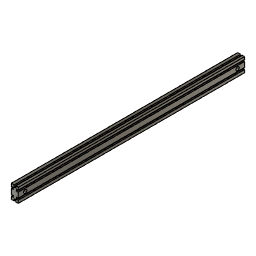
clearbot v9 (Autodesk Fusion 360 archive; units mm, degrees)
design "40X80X1300_AlBar"
Autodesk Fusion 360 part; units mm, degrees
sketch "Sketch1" plane through (0, 0, 0) normal (0, 1, 0) x (1, 0, 0)
  line L0 (20, -40) -> (-20, 40) construction
  line L1 (-20, -40) -> (20, 40) construction
  line L2 (5, 29) -> (-5, 29)
  line L3 (-5, 29) -> (-5, 39)
  line L4 (5, 39) -> (5, 29)
  line L5 (5, 29) -> (-5, 39) construction
  line L6 (-5, 29) -> (5, 39) construction
  line L7 (-4, 39) -> (-4, 40)
  line L8 (4, 39) -> (4, 40)
  line L9 (-19, 25) -> (-9, 25)
  line L10 (-9, 25) -> (-9, 15)
  line L11 (-9, 15) -> (-19, 15)
  line L12 (19, 25) -> (9, 25)
  line L13 (9, 25) -> (9, 15)
  line L14 (9, 15) -> (19, 15)
  line L15 (-20, 16) -> (-19, 16)
  line L16 (-19, 24) -> (-20, 24)
  line L17 (19, 16) -> (20, 16)
  line L18 (20, 24) -> (19, 24)
  line L19 (-20, 24) -> (-20, 40)
  line L20 (-19, 15) -> (-19, 16)
  line L21 (-19, 24) -> (-19, 25)
  line L22 (19, 15) -> (19, 16)
  line L23 (19, 24) -> (19, 25)
  line L24 (-20, 40) -> (-4, 40)
  line L25 (4, 40) -> (20, 40)
  line L26 (-5, 39) -> (-4, 39)
  line L27 (4, 39) -> (5, 39)
  line L28 (20, 40) -> (20, 24)
  line L29 (1.75, 0) -> (22.5, 0)
  line L30 (-19, -24) -> (-20, -24)
  line L31 (-19, -24) -> (-19, -25)
  line L32 (-19, -25) -> (-9, -25)
  line L33 (-20, -16) -> (-19, -16)
  line L34 (-19, -15) -> (-19, -16)
  line L35 (-9, -15) -> (-19, -15)
  line L36 (-9, -25) -> (-9, -15)
  line L37 (-4, -39) -> (-4, -40)
  line L38 (-5, -39) -> (-4, -39)
  line L39 (-5, -29) -> (-5, -39)
  line L40 (5, -29) -> (-5, -29)
  line L41 (5, -39) -> (5, -29)
  line L42 (4, -39) -> (5, -39)
  line L43 (4, -39) -> (4, -40)
  line L44 (20, -24) -> (19, -24)
  line L45 (19, -24) -> (19, -25)
  line L46 (19, -25) -> (9, -25)
  line L47 (9, -25) -> (9, -15)
  line L48 (9, -15) -> (19, -15)
  line L49 (19, -15) -> (19, -16)
  line L50 (19, -16) -> (20, -16)
  line L51 (-20, -40) -> (-20, -24)
  line L52 (-20, -16) -> (-20, 16)
  line L53 (20, 16) -> (20, -16)
  line L54 (20, -24) -> (20, -40)
  line L55 (20, -40) -> (4, -40)
  line L56 (-4, -40) -> (-20, -40)
  point P0 (0, 34)
  dimension "d20" = 40
  dimension "d21" = 80
  dimension "d22" = 10
  dimension "d23" = 10
  dimension "d24" = 20
  dimension "d25" = 16
  dimension "d26" = 16
  dimension "d27" = 1
  dimension "d28" = 15
  dimension "d29" = 15
  dimension "d30" = 10
  dimension "d31" = 10
  dimension "d32" = 10
  dimension "d33" = 10
  dimension "d34" = 16
  dimension "d35" = 8
  dimension "d36" = 1
  dimension "d37" = 16
  dimension "d38" = 8
  dimension "d39" = 1
  constraint horizontal L55
  constraint perpendicular L51 L55
  constraint parallel L24 L55
  constraint parallel L28 L51
  constraint coincident L0 origin
  constraint coincident L1 origin
  constraint horizontal L2
  constraint perpendicular L2 L3
  constraint parallel L2 L26
  constraint parallel L3 L4
  constraint coincident L5 P0
  constraint coincident L6 P0
  constraint perpendicular L7 L24
  constraint coincident L8.start L26
  constraint coincident L8.end L24
  constraint perpendicular L8 L24
  constraint horizontal L9
  constraint vertical L10
  constraint horizontal L11
  constraint vertical L20
  constraint horizontal L12
  constraint vertical L13
  constraint horizontal L14
  constraint vertical L22
  constraint perpendicular L15 L20
  constraint coincident L16.start L20
  constraint coincident L16.end L51
  constraint perpendicular L16 L51
  constraint coincident L17.end L28
  constraint perpendicular L17 L28
  constraint coincident L18.end L22
  constraint perpendicular L18 L22
  constraint collinear L19 L51
  constraint collinear L20 L21
  constraint collinear L22 L23
  constraint collinear L24 L25
  constraint collinear L26 L27
  constraint collinear L28 L53
  constraint symmetric L2.start L29 L40.start
  constraint symmetric L2.end L29 L39.start
  constraint symmetric L3.end L29 L38.start
  constraint symmetric L4.start L29 L41.start
  constraint symmetric L7.start L29 L37.start
  constraint symmetric L7.end L29 L37.end
  constraint symmetric L8.start L29 L42.start
  constraint symmetric L8.end L29 L43.end
  constraint symmetric L9.start L29 L31.end
  constraint symmetric L9.end L29 L32.end
  constraint symmetric L10.end L29 L35.start
  constraint symmetric L11.end L29 L34.start
  constraint symmetric L12.start L29 L45.end
  constraint symmetric L12.end L29 L46.end
  constraint symmetric L13.end L29 L47.end
  constraint symmetric L14.end L29 L48.end
  constraint symmetric L15.start L29 L33.start
  constraint symmetric L15.end L29 L33.end
  constraint symmetric L16.start L29 L30.start
  constraint symmetric L16.end L29 L30.end
  constraint symmetric L17.start L29 L49.end
  constraint symmetric L17.end L29 L50.end
  constraint symmetric L18.start L29 L44.start
  constraint symmetric L18.end L29 L44.end
  constraint collinear L51 L52
  constraint collinear L53 L54
  constraint collinear L55 L56
  measures "d20" distance of L0.start L1.start
  measures "d21" distance of L0.start L1.end
  measures "d22" distance of L2.start L2.end
  measures "d23" distance of L2.start L4.start
  measures "d24" horizontal distance of L0.end P0
  measures "d25" distance of L0.end L7.end
  measures "d26" distance of L1.end L8.end
  measures "d27" distance of L8.start L8.end
  measures "d28" vertical distance of L0.end L9.start
  measures "d29" vertical distance of L1.end L12.start
  measures "d30" distance of L9.end L10.end
  measures "d31" distance of L9.start L9.end
  measures "d32" distance of L12.start L12.end
  measures "d33" distance of L12.end L13.end
  measures "d34" distance of L1.end L18.start
  measures "d35" distance of L17 L18.start
  measures "d36" distance of L18.start L18.end
  measures "d37" distance of L0.end L16.end
  measures "d38" distance of L15 L16
  measures "d39" distance of L16.start L16.end
extrude "Extrude1" add sketch "Sketch1" along normal blind 1300
sketch "Sketch2" plane through (20, 0, 0) normal (1, 0, 0) x (0, 1, 0)
  line L0 (0, 16) -> (0, -16)
  line L1 (0, -16) -> (1300, -16)
  line L2 (1300, -16) -> (1300, 16)
  line L3 (1300, 16) -> (0, 16)
  circle A0 centre (40, 0) radius 10
  circle A1 centre (1260, 0) radius 10
  dimension "d42" = 20
  dimension "d45" = 20
  dimension "d48" = 40
  dimension "d49" = 40
  measures "d42" diameter of A0
  measures "d45" diameter of A1
  measures "d48" distance of origin A0.centre
  measures "d49" distance of L2 A1.centre
extrude "Extrude2" cut sketch "Sketch2" against normal blind 40 contours A0
extrude "Extrude3" cut sketch "Sketch2" against normal blind 35 contours A1
